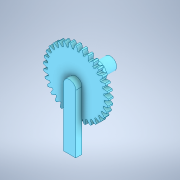
# Autodesk Inventor part: outerGear
Saved by Autodesk Inventor 2020.1 (Build 241239000, 239)
## iProperties
Created: 2020-01-18
Part Number: outerGear
Material: Generic
Document SubType Name: Modeling
Designer: Ali
Density: 1 g/cm^3
Appearance: Default
Author: Ali
Autodesk Inventor part; units mm, degrees
ref_plane "YZ Plane" through (0, 0, 0) normal (1, 0, 0) x (0, 1, 0)
ref_plane "XZ Plane" through (0, 0, 0) normal (0, 1, 0) x (-1, 0, 0)
ref_plane "XY Plane" through (0, 0, 0) normal (0, 0, 1) x (1, 0, 0)
sketch "Sketch1" plane through (0, 0, 0) normal (0, 0, 1) x (1, 0, 0)
  circle A0 centre (0, 0) radius 12.5
  dimension "d0" = 25
  constraints: 1 centre point, 1 coincident
  measures "d0" diameter of A0
extrude "Extrusion1" add sketch "Sketch1" along normal blind 2
sketch "Sketch2" plane through (0, 0, 2) normal (0, 0, 1) x (1, 0, 0)
  circle A0 centre (0, 0) radius 2.5
  dimension "d3" = 5
  constraints: 1 centre point, 1 coincident
  measures "d3" diameter of A0
extrude "Extrusion2" add sketch "Sketch2" along normal blind 9
ref_plane "Work Plane1" through (0, 0, 9) normal (0, 0, 1) x (1, 0, 0)
sketch "Sketch5" plane through (0, 0, 9) normal (0, 0, 1) x (1, 0, 0)
  circle A0 centre (0, 0) radius 2.5 projected
  circle A1 centre (0, 0) radius 3.5
  dimension "d18" = 1
  constraints: 1 centre point
  measures "d18" radial gap between concentric circles of A0 A1
extrude "Extrusion7" add sketch "Sketch5" against normal blind 1
sketch "Sketch6" plane through (0, 0, 0) normal (0, 0, -1) x (-1, 0, 0)
  circle A0 centre (0, 0) radius 12.5 projected
  circle A1 centre (0, 0) radius 2.5
  line L0 (-2.5, 0) -> (2.5, 0)
  line L1 (2.5, 0) -> (2.5, -23.6726)
  line L2 (2.5, -23.6726) -> (-2.5, -23.6726)
  line L3 (-2.5, -23.6726) -> (-2.5, 0)
  circle A2 centre (0, 0) radius 2.5 projected
  point P0 (2.5, 0)
  dimension "d23" = 5
  dimension "d24" = 5
  dimension "d25" = 23.6726
  constraints: 8 end point, 2 parallel, 1 centre point, 1 coincident, 1 horizontal, 1 horizontal alignment, 1 perpendicular, 1 other
  measures "d23" diameter of A1
  measures "d24" distance of L0.start L0.end
  measures "d25" distance of L0.end L1.end
extrude "Extrusion8" add sketch "Sketch6" along normal blind 2.5 contours L3 A1 L1 A0 | A0 L1 L2 L3 | L0 A1 | A1 L0 picked at (0.1004, -9.1418)
sketch "Sketch8" plane through (0, 0, 11) normal (0, 0, 1) x (1, 0, 0)
  circle A0 centre (0, 0) radius 2.5 projected
extrude "Extrusion10" add sketch "Sketch8" along normal blind 3
sketch "Sketch10" plane through (0, 0, 0) normal (0, 0, -1) x (-1, 0, 0)
  line L0 (2.5, 0) -> (2.5, -12.2474) projected
  arc A0 (2.5, -12.2474) -> (-2.5, -12.2474) centre (0, 0) ccw projected
  line L1 (-2.5, -12.2474) -> (-2.5, 0) projected
  arc A1 (2.5, 0) -> (-2.5, 0) centre (0, 0) ccw projected
  arc A2 (-2.5, -12.2474) -> (2.5, -12.2474) centre (0, 0) ccw projected
extrude "Extrusion12" cut sketch "Sketch10" against normal blind 2
sketch "Sketch11" plane through (0, 0, 2) normal (0, 0, -1) x (-1, 0, 0)
  arc A0 (-2.7899, 12.8251) -> (-2.9602, 11.0478) centre (4.8357, 11.1975) ccw
  arc A1 (-2.9602, 11.0478) -> (-3.4826, 10.8944) centre (0, 0) ccw
  arc A2 (-3.4826, 10.8944) -> (-4.5867, 12.2975) centre (-10.1219, 6.8055) ccw
  arc A3 (-4.5867, 12.2975) -> (-5.1667, 12.0653) centre (0, 0) ccw
  arc A4 (-5.1667, 12.0653) -> (-4.9976, 10.2879) centre (2.6292, 11.9103) ccw
  arc A5 (-4.9976, 10.2879) -> (-5.4814, 10.0385) centre (0, 0) ccw
  arc A6 (-5.4814, 10.0385) -> (-6.8311, 11.2072) centre (-11.2269, 4.767) ccw
  arc A7 (-6.8311, 11.2072) -> (-7.3567, 10.8695) centre (0, 0) ccw
  arc A8 (-7.3567, 10.8695) -> (-6.8542, 9.1562) centre (0.3276, 12.1926) ccw
  arc A9 (-6.8542, 9.1562) -> (-7.2821, 8.8197) centre (0, 0) ccw
  arc A10 (-7.2821, 8.8197) -> (-8.8287, 9.7119) centre (-11.9262, 2.5561) ccw
  arc A11 (-8.8287, 9.7119) -> (-9.2808, 9.2808) centre (0, 0) ccw
  arc A12 (-9.2808, 9.2808) -> (-8.4632, 7.6936) centre (-1.9857, 12.0343) ccw
  arc A13 (-8.4632, 7.6936) -> (-8.8197, 7.2821) centre (0, 0) ccw
  arc A14 (-8.8197, 7.2821) -> (-10.5071, 7.8655) centre (-12.1944, 0.2529) ccw
  arc A15 (-10.5071, 7.8655) -> (-10.8695, 7.3567) centre (0, 0) ccw
  arc A16 (-10.8695, 7.3567) -> (-9.7663, 5.9529) centre (-4.2274, 11.441) ccw
  arc A17 (-9.7663, 5.9529) -> (-10.0385, 5.4814) centre (0, 0) ccw
  arc A18 (-10.0385, 5.4814) -> (-11.8058, 5.7349) centre (-12.0219, -2.0595) ccw
  arc A19 (-11.8058, 5.7349) -> (-12.0653, 5.1667) centre (0, 0) ccw
  arc A20 (-12.0653, 5.1667) -> (-10.7164, 3.997) centre (-6.3162, 10.4342) ccw
  arc A21 (-10.7164, 3.997) -> (-10.8944, 3.4826) centre (0, 0) ccw
  arc A22 (-10.8944, 3.4826) -> (-12.6778, 3.397) centre (-11.4149, -4.2974) ccw
  arc A23 (-12.6778, 3.397) -> (-12.8251, 2.7899) centre (0, 0) ccw
  arc A24 (-12.8251, 2.7899) -> (-11.2791, 1.8967) centre (-8.1767, 9.0503) ccw
  arc A25 (-11.2791, 1.8967) -> (-11.3566, 1.3578) centre (0, 0) ccw
  arc A26 (-11.3566, 1.3578) -> (-13.0916, 0.9363) centre (-10.3953, -6.3801) ccw
  arc A27 (-13.0916, 0.9363) -> (-13.1213, 0.3123) centre (0, 0) ccw
  arc A28 (-13.1213, 0.3123) -> (-11.4343, -0.2722) centre (-9.7418, 7.3393) ccw
  arc A29 (-11.4343, -0.2722) -> (-11.4084, -0.8159) centre (0, 0) ccw
  arc A30 (-11.4084, -0.8159) -> (-13.0322, -1.5582) centre (-9, -8.2321) ccw
  arc A31 (-13.0322, -1.5582) -> (-12.9433, -2.1765) centre (0, 0) ccw
  arc A32 (-12.9433, -2.1765) -> (-11.1761, -2.4312) centre (-10.9547, 5.363) ccw
  arc A33 (-11.1761, -2.4312) -> (-11.0478, -2.9602) centre (0, 0) ccw
  arc A34 (-11.0478, -2.9602) -> (-12.5018, -3.9964) centre (-7.2794, -9.7866) ccw
  arc A35 (-12.5018, -3.9964) -> (-12.2975, -4.5867) centre (0, 0) ccw
  arc A36 (-12.2975, -4.5867) -> (-10.514, -4.5024) centre (-11.7717, 3.1929) ccw
  arc A37 (-10.514, -4.5024) -> (-10.2879, -4.9976) centre (0, 0) ccw
  arc A38 (-10.2879, -4.9976) -> (-11.5195, -6.2901) centre (-5.2958, -10.9874) ccw
  arc A39 (-11.5195, -6.2901) -> (-11.2072, -6.8311) centre (0, 0) ccw
  arc A40 (-11.2072, -6.8311) -> (-9.472, -6.4108) centre (-12.1632, 0.9074) ccw
  arc A41 (-9.472, -6.4108) -> (-9.1562, -6.8542) centre (0, 0) ccw
  arc A42 (-9.1562, -6.8542) -> (-10.1209, -8.3566) centre (-3.1207, -11.791) ccw
  arc A43 (-10.1209, -8.3566) -> (-9.7119, -8.8287) centre (0, 0) ccw
  arc A44 (-9.7119, -8.8287) -> (-8.0875, -8.0875) centre (-12.1151, -1.4109) ccw
  arc A45 (-8.0875, -8.0875) -> (-7.6936, -8.4632) centre (0, 0) ccw
  arc A46 (-7.6936, -8.4632) -> (-8.3566, -10.1209) centre (-0.8328, -12.1685) ccw
  arc A47 (-8.3566, -10.1209) -> (-7.8655, -10.5071) centre (0, 0) ccw
  arc A48 (-7.8655, -10.5071) -> (-6.4108, -9.472) centre (-11.6292, -3.6782) ccw
  arc A49 (-6.4108, -9.472) -> (-5.9529, -9.7663) centre (0, 0) ccw
  arc A50 (-5.9529, -9.7663) -> (-6.2901, -11.5195) centre (1.4851, -12.1063) ccw
  arc A51 (-6.2901, -11.5195) -> (-5.7349, -11.8058) centre (0, 0) ccw
  arc A52 (-5.7349, -11.8058) -> (-4.5024, -10.514) centre (-10.7229, -5.8126) ccw
  arc A53 (-4.5024, -10.514) -> (-3.997, -10.7164) centre (0, 0) ccw
  arc A54 (-3.997, -10.7164) -> (-3.9964, -12.5018) centre (3.7494, -11.6064) ccw
  arc A55 (-3.9964, -12.5018) -> (-3.397, -12.6778) centre (0, 0) ccw
  arc A56 (-3.397, -12.6778) -> (-2.4312, -11.1761) centre (-9.4291, -7.7368) ccw
  arc A57 (-2.4312, -11.1761) -> (-1.8967, -11.2791) centre (0, 0) ccw
  arc A58 (-1.8967, -11.2791) -> (-1.5582, -13.0322) centre (5.8782, -10.6871) ccw
  arc A59 (-1.5582, -13.0322) -> (-0.9363, -13.0916) centre (0, 0) ccw
  arc A60 (-0.9363, -13.0916) -> (-0.2722, -11.4343) centre (-7.7945, -9.3815) ccw
  arc A61 (-0.2722, -11.4343) -> (0.2722, -11.4343) centre (0, 0) ccw
  arc A62 (0.2722, -11.4343) -> (0.9363, -13.0916) centre (7.7945, -9.3815) ccw
  arc A63 (0.9363, -13.0916) -> (1.5582, -13.0322) centre (0, 0) ccw
  arc A64 (1.5582, -13.0322) -> (1.8967, -11.2791) centre (-5.8782, -10.6871) ccw
  arc A65 (1.8967, -11.2791) -> (2.4312, -11.1761) centre (0, 0) ccw
  arc A66 (2.4312, -11.1761) -> (3.397, -12.6778) centre (9.4291, -7.7368) ccw
  arc A67 (3.397, -12.6778) -> (3.9964, -12.5018) centre (0, 0) ccw
  arc A68 (3.9964, -12.5018) -> (3.997, -10.7164) centre (-3.7494, -11.6064) ccw
  arc A69 (3.997, -10.7164) -> (4.5024, -10.514) centre (0, 0) ccw
  arc A70 (4.5024, -10.514) -> (5.7349, -11.8058) centre (10.7229, -5.8126) ccw
  arc A71 (5.7349, -11.8058) -> (6.2901, -11.5195) centre (0, 0) ccw
  arc A72 (6.2901, -11.5195) -> (5.9529, -9.7663) centre (-1.4851, -12.1063) ccw
  arc A73 (5.9529, -9.7663) -> (6.4108, -9.472) centre (0, 0) ccw
  arc A74 (6.4108, -9.472) -> (7.8655, -10.5071) centre (11.6292, -3.6782) ccw
  arc A75 (7.8655, -10.5071) -> (8.3566, -10.1209) centre (0, 0) ccw
  arc A76 (8.3566, -10.1209) -> (7.6936, -8.4632) centre (0.8328, -12.1685) ccw
  arc A77 (7.6936, -8.4632) -> (8.0875, -8.0875) centre (0, 0) ccw
  arc A78 (8.0875, -8.0875) -> (9.7119, -8.8287) centre (12.1151, -1.4109) ccw
  arc A79 (9.7119, -8.8287) -> (10.1209, -8.3566) centre (0, 0) ccw
  arc A80 (10.1209, -8.3566) -> (9.1562, -6.8542) centre (3.1207, -11.791) ccw
  arc A81 (9.1562, -6.8542) -> (9.472, -6.4108) centre (0, 0) ccw
  arc A82 (9.472, -6.4108) -> (11.2072, -6.8311) centre (12.1632, 0.9074) ccw
  arc A83 (11.2072, -6.8311) -> (11.5195, -6.2901) centre (0, 0) ccw
  arc A84 (11.5195, -6.2901) -> (10.2879, -4.9976) centre (5.2958, -10.9874) ccw
  arc A85 (10.2879, -4.9976) -> (10.514, -4.5024) centre (0, 0) ccw
  arc A86 (10.514, -4.5024) -> (12.2975, -4.5867) centre (11.7717, 3.1929) ccw
  arc A87 (12.2975, -4.5867) -> (12.5018, -3.9964) centre (0, 0) ccw
  arc A88 (12.5018, -3.9964) -> (11.0478, -2.9602) centre (7.2794, -9.7866) ccw
  arc A89 (11.0478, -2.9602) -> (11.1761, -2.4312) centre (0, 0) ccw
  arc A90 (11.1761, -2.4312) -> (12.9433, -2.1765) centre (10.9547, 5.363) ccw
  arc A91 (12.9433, -2.1765) -> (13.0322, -1.5582) centre (0, 0) ccw
  arc A92 (13.0322, -1.5582) -> (11.4084, -0.8159) centre (9, -8.2321) ccw
  arc A93 (11.4084, -0.8159) -> (11.4343, -0.2722) centre (0, 0) ccw
  arc A94 (11.4343, -0.2722) -> (13.1213, 0.3123) centre (9.7418, 7.3393) ccw
  arc A95 (13.1213, 0.3123) -> (13.0916, 0.9363) centre (0, 0) ccw
  arc A96 (13.0916, 0.9363) -> (11.3566, 1.3578) centre (10.3953, -6.3801) ccw
  arc A97 (11.3566, 1.3578) -> (11.2791, 1.8967) centre (0, 0) ccw
  arc A98 (11.2791, 1.8967) -> (12.8251, 2.7899) centre (8.1767, 9.0503) ccw
  arc A99 (12.8251, 2.7899) -> (12.6778, 3.397) centre (0, 0) ccw
  arc A100 (12.6778, 3.397) -> (10.8944, 3.4826) centre (11.4149, -4.2974) ccw
  arc A101 (10.8944, 3.4826) -> (10.7164, 3.997) centre (0, 0) ccw
  arc A102 (10.7164, 3.997) -> (12.0653, 5.1667) centre (6.3162, 10.4342) ccw
  arc A103 (12.0653, 5.1667) -> (11.8058, 5.7349) centre (0, 0) ccw
  arc A104 (11.8058, 5.7349) -> (10.0385, 5.4814) centre (12.0219, -2.0595) ccw
  arc A105 (10.0385, 5.4814) -> (9.7663, 5.9529) centre (0, 0) ccw
  arc A106 (9.7663, 5.9529) -> (10.8695, 7.3567) centre (4.2274, 11.441) ccw
  arc A107 (10.8695, 7.3567) -> (10.5071, 7.8655) centre (0, 0) ccw
  arc A108 (10.5071, 7.8655) -> (8.8197, 7.2821) centre (12.1944, 0.2529) ccw
  arc A109 (8.8197, 7.2821) -> (8.4632, 7.6936) centre (0, 0) ccw
  arc A110 (8.4632, 7.6936) -> (9.2808, 9.2808) centre (1.9857, 12.0343) ccw
  arc A111 (9.2808, 9.2808) -> (8.8287, 9.7119) centre (0, 0) ccw
  arc A112 (8.8287, 9.7119) -> (7.2821, 8.8197) centre (11.9262, 2.5561) ccw
  arc A113 (7.2821, 8.8197) -> (6.8542, 9.1562) centre (0, 0) ccw
  arc A114 (6.8542, 9.1562) -> (7.3567, 10.8695) centre (-0.3276, 12.1926) ccw
  arc A115 (7.3567, 10.8695) -> (6.8311, 11.2072) centre (0, 0) ccw
  arc A116 (6.8311, 11.2072) -> (5.4814, 10.0385) centre (11.2269, 4.767) ccw
  arc A117 (5.4814, 10.0385) -> (4.9976, 10.2879) centre (0, 0) ccw
  arc A118 (4.9976, 10.2879) -> (5.1667, 12.0653) centre (-2.6292, 11.9103) ccw
  arc A119 (5.1667, 12.0653) -> (4.5867, 12.2975) centre (0, 0) ccw
  arc A120 (4.5867, 12.2975) -> (3.4826, 10.8944) centre (10.1219, 6.8055) ccw
  arc A121 (3.4826, 10.8944) -> (2.9602, 11.0478) centre (0, 0) ccw
  arc A122 (2.9602, 11.0478) -> (2.7899, 12.8251) centre (-4.8357, 11.1975) ccw
  arc A123 (2.7899, 12.8251) -> (2.1765, 12.9433) centre (0, 0) ccw
  arc A124 (2.1765, 12.9433) -> (1.3578, 11.3566) centre (8.651, 8.5981) ccw
  arc A125 (1.3578, 11.3566) -> (0.8159, 11.4084) centre (0, 0) ccw
  arc A126 (0.8159, 11.4084) -> (0.3123, 13.1213) centre (-6.8675, 10.0799) ccw
  arc A127 (0.3123, 13.1213) -> (-0.3123, 13.1213) centre (0, 0) ccw
  arc A128 (-0.3123, 13.1213) -> (-0.8159, 11.4084) centre (6.8675, 10.0799) ccw
  arc A129 (-0.8159, 11.4084) -> (-1.3578, 11.3566) centre (0, 0) ccw
  arc A130 (-1.3578, 11.3566) -> (-2.1765, 12.9433) centre (-8.651, 8.5981) ccw
  arc A131 (-2.1765, 12.9433) -> (-2.7899, 12.8251) centre (0, 0) ccw
  constraints: 264 point on circle, 132 centre point
extrude "Extrusion13" add sketch "Sketch11" along normal blind 2
equation "\"d0\" = OG_gearDiameter"
equation "\"d1\" = OG_gearThickness"
equation "\"d3\" = OG_shaftDiameter"
equation "\"d4\" = OG_shaftLength"
equation "\"d19\" = OG_skirtThickness"
equation "\"Wheel_Related_W_\" = 0"
equation "\"W_innerDepth\" = 4"
equation "\"W_wallThickness\" = 2"
equation "\"W_holesClearance\" = 0.3"
equation "\"W_outerGearHoleDiameter\" = 5.3"
equation "\"W_innerGearHoleDiameter\" = 10.1"
equation "\"TempSpotReserved7\" = 0"
equation "\"TempSpotReserved8\" = 0"
equation "\"TempSpotReserved9\" = 0"
equation "\"TempSpotReserved10\" = 0"
equation "\"TempSpotReserved11\" = 0"
equation "\"TempSpotReserved12\" = 0"
equation "\"TempSpotReserved13\" = 0"
equation "\"TempSpotReserved14\" = 0"
equation "\"TempSpotReserved15\" = 0"
equation "\"TempSpotReserved16\" = 0"
equation "\"TempSpotReserved17\" = 0"
equation "\"TempSpotReserved18\" = 0"
equation "\"TempSpotReserved19\" = 0"
equation "\"TempSpotReserved20\" = 0"
equation "\"Inner_Gear_Related_IG_\" = 0"
equation "\"IG_shaftDiameter\" = 7.5"
equation "\"IG_shaftLength\" = 17"
equation "\"IG_gearThickness\" = 2"
equation "\"TempSpotReserved25\" = 0"
equation "\"TempSpotReserved26\" = 0"
equation "\"TempSpotReserved27\" = 0"
equation "\"TempSpotReserved28\" = 0"
equation "\"TempSpotReserved29\" = 0"
equation "\"TempSpotReserved30\" = 0"
equation "\"TempSpotReserved31\" = 0"
equation "\"TempSpotReserved32\" = 0"
equation "\"TempSpotReserved33\" = 0"
equation "\"TempSpotReserved34\" = 0"
equation "\"TempSpotReserved35\" = 0"
equation "\"TempSpotReserved36\" = 0"
equation "\"TempSpotReserved37\" = 0"
equation "\"TempSpotReserved38\" = 0"
equation "\"TempSpotReserved39\" = 0"
equation "\"TempSpotReserved40\" = 0"
equation "\"Outer_Gear_Related_OG_\" = 0"
equation "\"OG_distanceFromCenter\" = 22.5"
equation "\"OG_shaftDiameter\" = 5"
equation "\"OG_gearDiameter\" = 25"
equation "\"OG_shaftLength\" = 9"
equation "\"OG_gearThickness\" = 2"
equation "\"TempSpotReserved47\" = 0"
equation "\"TempSpotReserved48\" = 0"
equation "\"TempSpotReserved49\" = 0"
equation "\"TempSpotReserved50\" = 0"
equation "\"TempSpotReserved51\" = 0"
equation "\"TempSpotReserved52\" = 0"
equation "\"TempSpotReserved53\" = 0"
equation "\"TempSpotReserved54\" = 0"
equation "\"TempSpotReserved55\" = 0"
equation "\"TempSpotReserved56\" = 0"
equation "\"TempSpotReserved57\" = 0"
equation "\"TempSpotReserved58\" = 0"
equation "\"TempSpotReserved59\" = 0"
equation "\"TempSpotReserved60\" = 0"
equation "\"Leg_Extensions_Related_LE_\" = 0"
equation "\"LE_baseDiameter\" = 5"
equation "\"LE_maxLength\" = 23.67256"
equation "\"LE_thickness\" = 2.5"
equation "\"IG_ratioToOuterGear\" = 1.25"
equation "\"B_bearingThickness\" = 1"
equation "\"TempSpotReserved43\" = 0"
equation "\"TempSpotReserved45\" = 0"
equation "\"Thisisatest\" = 25.4"
equation "\"TempSpotReserved46\" = 0"
equation "\"TempSpotReserved44\" = 0"
equation "\"LE_offsetAboveOuterGear\" = 0"
equation "\"Bearing_Related_B_\" = 0"
equation "\"TempSpotReserved42\" = 0"
equation "\"OG_skirtOffset\" = 5"
equation "\"OG_skirtThickness\" = 1"
equation "\"IG_skirtThickness\" = 2"
equation "\"IG_extentionLength\" = 19.5"
equation "\"IG_extentionThickness\" = 3"
equation "\"IG_slitWidth\" = 4"
equation "\"IG_slitlength\" = 8"
equation "\"IG_slitDistanceFromCenterHole\" = 7"
equation "\"IG_slitClearance\" = 0.2"
equation "\"Reserved_10\" = 0"
equation "\"Reserved_9\" = 0"
equation "\"Reserved_11\" = 0"
equation "\"Reserved_12\" = 0"
equation "\"Reserved_8\" = 0"
equation "\"Reserved_7\" = 0"
equation "\"Reserved_26\" = 0"
equation "\"Reserved_20\" = 0"
equation "\"Reserved_22\" = 0"
equation "\"Reserved_23\" = 0"
equation "\"Reserved_25\" = 0"
equation "\"Reserved_24\" = 0"
equation "\"Reserved_21\" = 0"
equation "\"Reserved_19\" = 0"
equation "\"Reserved_27\" = 0"
equation "\"Reserved_14\" = 0"
equation "\"Reserved_15\" = 0"
equation "\"Reserved_16\" = 0"
equation "\"Reserved_13\" = 0"
equation "\"Reserved_17\" = 0"
equation "\"Reserved_18\" = 0"
equation "\"Bearing_Related_BR_\" = 0"
equation "\"BR_bearingThickness\" = 1"
equation "\"Block_Related_BL_\" = 0"
equation "\"BL_width\" = 3.8"
equation "\"BL_length\" = 7.8"
equation "\"W_filletRadius\" = 0.25"
equation "\"W_extrutsionTaperAngle\" = 2deg"
equation "\"OG_protrudeDistance\" = 3"
equation "\"IG_dAxleCircleDiameter\" = 2"
equation "\"IG_dAxleShort\" = 1.5"
equation "\"IG_dAxleDepth\" = 5"
equation "\"IG_gearRatio\" = 1.25"
body "Solid1"
